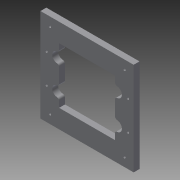
# Autodesk Inventor part: 300 mm core xy mount
Saved by Autodesk Inventor 2014 SP1 (Build 180222100, 222)
## iProperties
Created: 2014-09-28
Part Number: 300 mm core xy mount
Material: Generic
Document SubType Name: Modeling
Designer: Mon
Density: 1 g/cm^3
Appearance: Default
Author: Mon
Autodesk Inventor part; units mm, degrees
ref_plane "YZ Plane" through (0, 0, 0) normal (1, 0, 0) x (0, 1, 0)
ref_plane "XZ Plane" through (0, 0, 0) normal (0, 1, 0) x (-1, 0, 0)
ref_plane "XY Plane" through (0, 0, 0) normal (0, 0, 1) x (1, 0, 0)
sketch "Sketch1" plane through (0, 0, 0) normal (0, 1, 0) x (-1, 0, 0)
  line L0 (381.1955, 61.6323) -> (30.4817, 61.6323)
  line L1 (380.9912, 412.4092) -> (381.1955, 61.6323)
  line L2 (30.2774, 412.4092) -> (380.9912, 412.4092)
  line L3 (30.4817, 61.6323) -> (30.4817, 412.4092)
  arc A0 (0.1441, 15.9323) -> (16.1441, -0.0677) centre (16.1441, 15.9323) ccw
  line L4 (0.1817, 15.9323) -> (-0.0226, 429.4092)
  arc A1 (15.9774, 445.4092) -> (-0.0226, 429.4092) centre (15.9774, 429.4092) ccw
  line L5 (15.9774, 445.4092) -> (395.2912, 445.4092)
  arc A2 (411.2912, 429.4092) -> (395.2912, 445.4092) centre (395.2912, 429.4092) ccw
  line L6 (411.2912, 429.4092) -> (411.4955, 15.9323)
  arc A3 (395.4579, -0.0677) -> (411.4579, 15.9323) centre (395.4579, 15.9323) ccw
  line L7 (395.4579, -0.0677) -> (16.1441, -0.0677)
  arc A4 (21.4191, 6.4323) -> (25.1691, 6.4323) centre (23.2941, 6.4323) ccw
  line L8 (25.1691, 10.4323) -> (25.1691, 6.4323)
  arc A5 (25.1691, 10.4323) -> (21.4191, 10.4323) centre (23.2941, 10.4323) ccw
  line L9 (21.4191, 6.4323) -> (21.4191, 10.4323)
  arc A6 (52.4191, 6.4323) -> (56.1691, 6.4323) centre (54.2941, 6.4323) ccw
  line L10 (56.1691, 10.4323) -> (56.1691, 6.4323)
  arc A7 (56.1691, 10.4323) -> (52.4191, 10.4323) centre (54.2941, 10.4323) ccw
  line L11 (52.4191, 6.4323) -> (52.4191, 10.4323)
  arc A8 (21.4191, 37.4323) -> (25.1691, 37.4323) centre (23.2941, 37.4323) ccw
  line L12 (25.1691, 41.4323) -> (25.1691, 37.4323)
  arc A9 (25.1691, 41.4323) -> (21.4191, 41.4323) centre (23.2941, 41.4323) ccw
  line L13 (21.4191, 37.4323) -> (21.4191, 41.4323)
  arc A10 (52.4191, 37.4323) -> (56.1691, 37.4323) centre (54.2941, 37.4323) ccw
  line L14 (56.1691, 41.4323) -> (56.1691, 37.4323)
  arc A11 (56.1691, 41.4323) -> (52.4191, 41.4323) centre (54.2941, 41.4323) ccw
  line L15 (52.4191, 37.4323) -> (52.4191, 41.4323)
  arc A12 (26.7941, 21.9323) -> (50.7941, 21.9323) centre (38.7941, 21.9323) ccw
  line L16 (50.7941, 25.9323) -> (50.7941, 21.9323)
  arc A13 (50.7941, 25.9323) -> (26.7941, 25.9323) centre (38.7941, 25.9323) ccw
  line L17 (26.7941, 21.9323) -> (26.7941, 25.9323)
  arc A14 (355.464, 6.4323) -> (359.214, 6.4323) centre (357.339, 6.4323) ccw
  line L18 (359.214, 10.4323) -> (359.214, 6.4323)
  arc A15 (359.214, 10.4323) -> (355.464, 10.4323) centre (357.339, 10.4323) ccw
  line L19 (355.4329, 6.4323) -> (355.4329, 10.4323)
  arc A16 (386.4154, 6.4323) -> (390.1654, 6.4323) centre (388.2904, 6.3762) ccw
  arc A17 (386.4224, 37.4323) -> (390.1724, 37.4323) centre (388.2974, 37.4323) ccw
  line L20 (390.1724, 41.4323) -> (390.1724, 37.4323)
  arc A18 (390.1829, 41.4323) -> (386.4329, 41.4323) centre (388.3079, 41.4323) ccw
  line L21 (386.4224, 37.4323) -> (386.4224, 41.4323)
  arc A19 (355.4138, 37.4323) -> (359.1638, 37.4323) centre (357.2888, 37.4323) ccw
  line L22 (359.1638, 41.4323) -> (359.1638, 37.4323)
  arc A20 (359.1829, 41.4323) -> (355.4329, 41.4323) centre (357.3079, 41.4323) ccw
  line L23 (355.4138, 37.4323) -> (355.4138, 41.4323)
  arc A21 (360.7688, 21.9323) -> (384.7688, 21.9323) centre (372.7688, 21.9323) ccw
  line L24 (384.7688, 25.9323) -> (384.7688, 21.9323)
  arc A22 (384.8079, 25.9323) -> (360.8079, 25.9323) centre (372.8079, 25.9323) ccw
  line L25 (360.7688, 21.9323) -> (360.7688, 25.9323)
  circle A23 centre (50.2274, 420.4092) radius 2.1
  circle A24 centre (38.6274, 435.4092) radius 2.1
  circle A25 centre (372.6412, 435.4092) radius 2.1
  circle A26 centre (361.0412, 420.4092) radius 2.1
  circle A27 centre (25.8649, 417.9092) radius 1.6
  circle A28 centre (66.8649, 417.9092) radius 1.6
  circle A29 centre (205.6343, 417.9092) radius 1.6
  circle A30 centre (344.4037, 417.9092) radius 1.6
  circle A31 centre (385.4037, 417.9092) radius 1.6
  circle A32 centre (385.4037, 56.1323) radius 1
  circle A33 centre (344.4037, 56.1323) radius 1
  circle A34 centre (205.6343, 56.1323) radius 1
  circle A35 centre (66.8649, 56.1323) radius 1
  circle A36 centre (25.8649, 56.1323) radius 1
  arc A37 (390.1829, 10.4323) -> (386.4329, 10.4323) centre (388.3079, 10.4323) ccw
  line L26 (378.904, 179.3957) -> (32.2792, 179.3957)
  circle A38 centre (60.7292, 222.6707) radius 1.6
  circle A39 centre (60.7292, 258.4832) radius 1.6
  circle A40 centre (60.7292, 186.8582) radius 1.6
  circle A41 centre (350.454, 186.8582) radius 1.6
  circle A42 centre (350.454, 222.6707) radius 1.6
  circle A43 centre (350.454, 258.4832) radius 1.6
  circle A44 centre (49.9292, 185.7457) radius 1.6
  circle A45 centre (49.9292, 259.5957) radius 1.6
  circle A46 centre (361.254, 222.6707) radius 1.6
  line L27 (378.904, 265.9457) -> (378.904, 179.3957)
  line L28 (345.954, 256.4207) -> (345.954, 188.9207)
  line L29 (65.2292, 256.4207) -> (345.954, 256.4207)
  line L30 (65.2292, 188.9207) -> (65.2292, 256.4207)
  line L31 (345.954, 188.9207) -> (65.2292, 188.9207)
  line L32 (32.2792, 179.3957) -> (32.2792, 265.9457)
  line L33 (32.2792, 265.9457) -> (378.904, 265.9457)
  circle A47 centre (50.2292, 204.3707) radius 2.1
  circle A48 centre (360.954, 204.3707) radius 2.1
  circle A49 centre (360.954, 240.9707) radius 2.1
  circle A50 centre (50.2292, 240.9707) radius 2.1
  line L34 (224.6843, 203.6207) -> (186.5843, 203.6207)
  line L35 (224.6843, 207.6798) -> (224.6843, 203.6207)
  arc A51 (226.0943, 209.1771) -> (224.6843, 207.6798) centre (226.1843, 207.6798) ccw
  arc A52 (226.0943, 209.1771) -> (226.0943, 216.1644) centre (225.8843, 212.6707) ccw
  arc A53 (224.6843, 217.6617) -> (226.0943, 216.1644) centre (226.1843, 217.6617) ccw
  arc A54 (226.0943, 229.1771) -> (224.6843, 227.6798) centre (226.1843, 227.6798) ccw
  arc A55 (226.0943, 229.1771) -> (226.0943, 236.1644) centre (225.8843, 232.6707) ccw
  arc A56 (224.6843, 237.6617) -> (226.0943, 236.1644) centre (226.1843, 237.6617) ccw
  line L36 (186.5843, 241.7207) -> (224.6843, 241.7207)
  line L37 (186.5843, 237.6617) -> (186.5843, 241.7207)
  arc A57 (185.1743, 236.1644) -> (186.5843, 237.6617) centre (185.0843, 237.6617) ccw
  arc A58 (185.1743, 236.1644) -> (185.1743, 229.1771) centre (185.3843, 232.6707) ccw
  arc A59 (186.5843, 227.6798) -> (185.1743, 229.1771) centre (185.0843, 227.6798) ccw
  arc A60 (185.1743, 216.1644) -> (186.5843, 217.6617) centre (185.0843, 217.6617) ccw
  arc A61 (185.1743, 216.1644) -> (185.1743, 209.1771) centre (185.3843, 212.6707) ccw
  arc A62 (186.5843, 207.6798) -> (185.1743, 209.1771) centre (185.0843, 207.6798) ccw
  line L38 (173.8843, 254.4207) -> (237.3843, 254.4207)
  line L39 (237.3843, 254.4207) -> (237.3843, 190.9207)
  line L40 (237.3843, 190.9207) -> (173.8843, 190.9207)
  line L41 (173.8843, 190.9207) -> (173.8843, 254.4207)
  circle A63 centre (180.2343, 196.8582) radius 0.875
  circle A64 centre (231.0343, 196.8582) radius 0.875
  circle A65 centre (231.0343, 248.4832) radius 0.875
  circle A66 centre (180.2343, 248.4832) radius 0.875
  circle A67 centre (177.8843, 232.6707) radius 0.875
  circle A68 centre (233.3843, 232.6707) radius 0.875
  circle A69 centre (233.3843, 212.6707) radius 0.875
  circle A70 centre (177.8843, 212.6707) radius 0.875
  line L42 (186.5843, 203.6207) -> (186.5843, 207.6798)
  line L43 (186.5843, 217.6617) -> (186.5843, 227.6798)
  line L44 (224.6843, 241.7207) -> (224.6843, 237.6617)
  line L45 (224.6843, 227.6798) -> (224.6843, 217.6617)
  line L46 (390.1829, 10.4323) -> (390.1829, 6.4239)
  line L47 (386.4329, 10.4323) -> (386.4329, 6.1144)
  circle A71 centre (136.8649, 56.1323) radius 1
  circle A72 centre (273.8973, 56.1323) radius 1
  circle A73 centre (274.4037, 417.9092) radius 1.6
  circle A74 centre (136.8649, 417.9092) radius 1.6
  point P0 (0, 0)
  constraints: 96 end point, 75 centre point, 73 point on circle, 1 point on line
extrude "Extrusion1" add sketch "Sketch1" along normal blind 4 contours L38 L39 L40 L41
body "Solid1"
